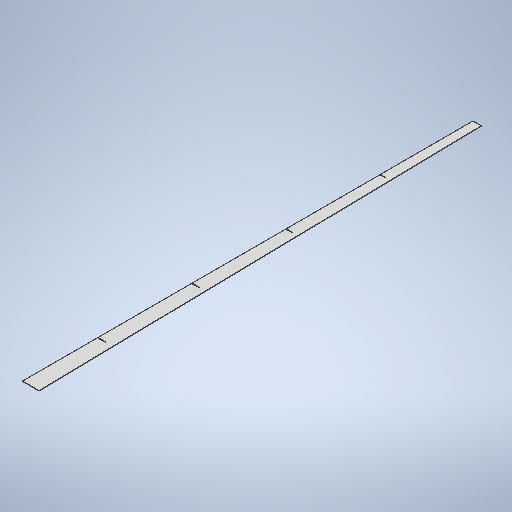
# Autodesk Inventor part: BSH 022 rib 2
Saved by Autodesk Inventor 2025 (Build 290162010, 162A)
## iProperties
Created: 2024-07-23
Part Number: BSH 022 rib 2
Material: Stainless Steel
Document SubType Name: Sheet Metal
Designer: admin
Density: 8 g/cm^3
Sheet Metal Rule: AISI304 3mm Die 32
Appearance: Default
Author: admin
Autodesk Inventor part; units mm, degrees
ref_plane "YZ Plane" through (0, 0, 0) normal (1, 0, 0) x (0, 1, 0)
ref_plane "XZ Plane" through (0, 0, 0) normal (0, 1, 0) x (-1, 0, 0)
ref_plane "XY Plane" through (0, 0, 0) normal (0, 0, 1) x (1, 0, 0)
sketch "Sketch1" plane through (0, 0, 0) normal (0, 0, 1) x (1, 0, 0)
  line L0 (1200, 2950) -> (-1200, 2950)
  line L1 (-1200, 2950) -> (-1200, 0)
  line L2 (-1200, 0) -> (1200, 0)
  line L3 (1200, 0) -> (1200, 2950)
  line L4 (1150, 2950) -> (1150, 0)
  line L5 (-1150, 0) -> (-1150, 2950) construction
  line L6 (0, 2950) -> (0, 50) construction
  line L7 (-1100, 200) -> (-950, 50)
  line L8 (-1200, 100) -> (-1100, 100)
  line L9 (-1100, 100) -> (-1100, 0)
  line L10 (-1100, 200) -> (-1150, 2950)
  arc A0 (-1100.4545, 224.9959) -> (-1082.3223, 182.3223) centre (-1100, 200) ccw
  arc A1 (-1082.3223, 182.3223) -> (-1100.4545, 224.9959) centre (-1100, 200) ccw construction
  line L11 (-1200, 255) -> (-1101, 255)
  line L12 (0, 50) -> (-950, 50)
  line L13 (0, 50) -> (0, 0)
  line L14 (1505.3449, -225.894) -> (355.3449, -225.894)
  dimension "d3" = 2400
  dimension "d4" = 2950
  dimension "d5" = 50
  dimension "d6" = 100
  dimension "d7" = 50
  dimension "d8" = 2695
  dimension "d9" = 135
  dimension "d10" = 950
  dimension "d11" = 1150
  dimension "d12" = 136.042
  dimension "d13" = 50
  dimension "d14" = 100
  dimension "d15" = 212.132
  dimension "d17" = 55
  dimension "d20" = 200
  measures "d3" distance of L3.start L1.end
  measures "d4" distance of L1.end L1.start
  measures "d5" diameter of A0
  measures "d6" distance of L8.start L8.end
  measures "d7" distance between parallel lines of L1 L5
  measures "d8" distance between parallel lines of L0 L11
  measures "d9" angle of L12 L7
  measures "d10" distance of L6.end L7.end
  measures "d11" distance of L14.start L14.end
  measures "d12" angle of L7 L10
  measures "d13" distance between parallel lines of L2 L12
  measures "d14" distance from line of L1 L10.start
  measures "d15" distance of L10.start L7.end
  measures "d17" vertical distance of L10.start L11.end
  measures "d20" distance from line of L2 A1.centre
extrude "Plate1" add sketch "Sketch1" along normal blind 3 contours L10 L11 L1 L0
sketch "Sketch2" plane through (0, 0, 3) normal (0, 0, 1) x (1, 0, 0)
  line L0 (-1101, 255) -> (-1200, 255) projected
  line L1 (-1150, 2950) -> (-1101, 255) projected
  line L2 (-1200, 2950) -> (-1150, 2950) projected
  line L3 (-1200, 255) -> (-1200, 2950) projected
  line L4 (-1101, 255) -> (-1150, 2950) projected
  line L5 (-1119.4769, 1271.232) -> (-1158.7453, 1270.5181) construction
  line L6 (-1158.7453, 1270.5181) -> (-1158.6871, 1267.3186)
  line L7 (-1158.6871, 1267.3186) -> (-1119.4188, 1268.0326) construction
  line L8 (-1150, 2950) -> (-1101, 255) projected
  line L9 (-1158.6871, 1267.3186) -> (-1200, 1266.5675)
  line L10 (-1158.7453, 1270.5181) -> (-1200, 1269.768)
  line L11 (-1200, 703.2744) -> (-1153.5904, 704.1182)
  line L12 (-1109.2386, 708.1251) -> (-1153.6486, 707.3177) construction
  line L13 (-1153.5904, 704.1182) -> (-1153.6486, 707.3177)
  line L14 (-1153.5904, 704.1182) -> (-1109.1805, 704.9256) construction
  line L15 (-1153.6486, 707.3177) -> (-1200, 706.4749)
  line L16 (-1200, 1829.8605) -> (-1163.7705, 1830.5193)
  line L17 (-1129.7153, 1834.339) -> (-1163.8287, 1833.7187) construction
  line L18 (-1163.7705, 1830.5193) -> (-1163.8287, 1833.7187)
  line L19 (-1163.8287, 1833.7187) -> (-1200, 1833.0611)
  line L20 (-1163.7705, 1830.5193) -> (-1129.6571, 1831.1395) construction
  line L21 (-1200, 2393.1536) -> (-1168.8606, 2393.7198)
  line L22 (-1139.9536, 2397.4459) -> (-1168.9188, 2396.9193) construction
  line L23 (-1168.8606, 2393.7198) -> (-1168.9188, 2396.9193)
  line L24 (-1168.8606, 2393.7198) -> (-1139.8954, 2394.2464) construction
  line L25 (-1168.9188, 2396.9193) -> (-1200, 2396.3542)
  point P0 (0, 0)
  point P1 (-1119.4188, 1268.0326)
  dimension "d24" = 3.2
  dimension "d32" = 450
  dimension "d33" = 3.2
  dimension "d34" = 46.4173
  dimension "d35" = 560
  dimension "d36" = 41.3197
  dimension "d37" = 560
  dimension "d38" = 3.2
  dimension "d39" = 36.2355
  dimension "d40" = 560
  dimension "d41" = 3.2
  dimension "d42" = 31.1445
  constraints: 40 end point, 13 parallel, 12 perpendicular, 2 collinear, 2 point on line, 18 other
  measures "d24" distance of L5.end L6.end
  measures "d32" distance from line of L11 L0.start
  measures "d33" distance between parallel lines of L12 L11
  measures "d34" distance of L11.start L11.end
  measures "d35" distance of L7.end L12.start
  measures "d36" distance of L9.end L6.end
  measures "d37" distance of L20.end L5.start
  measures "d38" distance between parallel lines of L16 L17
  measures "d39" distance of L16.start L16.end
  measures "d40" distance from line of L21 L17.start
  measures "d41" distance between parallel lines of L21 L22
  measures "d42" distance of L21.end L21.start
extrude "Extrusion1" cut sketch "Sketch2" against normal through all contours L3 L15 L13 L11 | L25 L23 L21 L3 | L3 L10 L6 L9 | L19 L18 L16 L3
equation "\"d11\" = d10 + d18"
equation "\"d14\" = d6"
equation "\"d32\" = Stringer1_hight"
equation "\"d35\" = Stringer1_step"
equation "\"d37\" = Stringer1_step"
equation "\"d40\" = Stringer1_step"
equation "\"d2\" = Thickness"
equation "\"BendReliefWidth\" = Thickness"
equation "\"BendReliefDepth\" = 0.5 * Thickness"
equation "\"CornerReliefSize\" = 4 * Thickness"
equation "\"MinimumRemnant\" = 2 * Thickness"
equation "\"TransitionRadius\" = BendRadius"
equation "\"JacobiRadiusSize\" = BendRadius"
equation "\"GapSize\" = Thickness"
equation "\"d18\" = d19"
equation "\"Stringer1_hight\" = 450"
equation "\"Stringer1_step\" = 560"
equation "\"Thickness\" = 3"
equation "\"BendRadius\" = 5"
equation "\"d19\" = 200"
body "Solid1"
